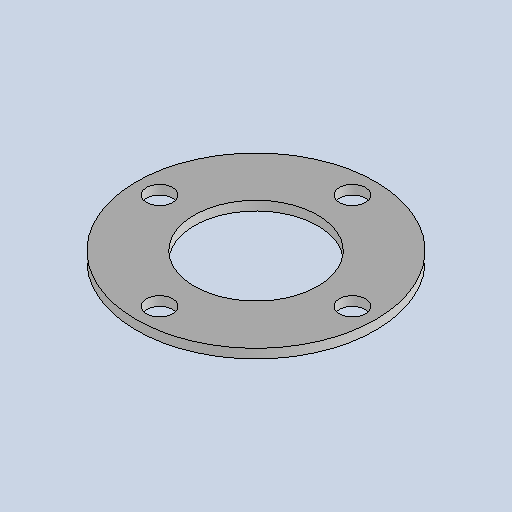
# Autodesk Inventor part: Flange DN 50
Saved by Autodesk Inventor 2025.1 (Build 291241020, 241B)
## iProperties
Created: 2025-05-22
Part Number: Flange DN 50
Material: Steel
Document SubType Name: Sheet Metal
Designer: user
Mass: 609.225 g
Surface Area: 315.809 cm^2
Volume: 77.6083 cm^3
Density: 7.85 g/cm^3
Sheet Metal Rule: AISI304 3mm Die 32
Sheet Metal Width: 155.000 mm
Sheet Metal Length: 155.000 mm
Sheet Metal Area: 24025.000 mm^2
Appearance: Default
Flat Pattern Width: 15.5 cm
Flat Pattern Length: 15.5 cm
Flat Pattern Area: 240.25 cm^2
Author: user
Autodesk Inventor part; units mm, degrees
ref_plane "YZ Plane" through (0, 0, 0) normal (1, 0, 0) x (0, 1, 0)
ref_plane "XZ Plane" through (0, 0, 0) normal (0, 1, 0) x (-1, 0, 0)
ref_plane "XY Plane" through (0, 0, 0) normal (0, 0, 1) x (1, 0, 0)
sketch "Sketch1" plane through (0, 0, 0) normal (0, 0, 1) x (1, 0, 0)
  circle A0 centre (0, 0) radius 77.5
  circle A1 centre (0, 0) radius 40
  dimension "d22" = 155
  dimension "d23" = 80
  measures "d22" diameter of A0
  measures "d23" diameter of A1
extrude "Plate1" add sketch "Sketch1" along normal blind 6
sketch "Sketch5" plane through (0, 0, 6) normal (0, 0, 1) x (1, 0, 0)
  circle A0 centre (0, -62.5) radius 8.5
  point P0 (0, 0)
  dimension "d24" = 62.5
  dimension "d25" = 17
  constraints: 1 centre point, 1 vertical alignment
  measures "d24" distance of A0.centre point (0, 0)
  measures "d25" diameter of A0
extrude "Cut1" cut sketch "Sketch5" against normal blind 6
pattern_circular "Circular Pattern1" count 4 over 360 about axis through (0, 0, 0) along (0, 0, 1) of "Cut1"
equation "\"d26\" = Thickness"
equation "\"d2\" = Thickness"
equation "\"BendReliefWidth\" = Thickness"
equation "\"BendReliefDepth\" = 0.5 * Thickness"
equation "\"CornerReliefSize\" = 4 * Thickness"
equation "\"MinimumRemnant\" = 2 * Thickness"
equation "\"TransitionRadius\" = BendRadius"
equation "\"JacobiRadiusSize\" = BendRadius"
equation "\"GapSize\" = Thickness"
equation "\"Thickness\" = 6"
equation "\"BendRadius\" = 5"
body "Solid1"
